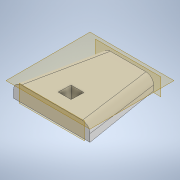
# Autodesk Inventor part: Botten
Saved by Autodesk Inventor 2021 (Build 250183000, 183)
## iProperties
Created: 2021-02-09
Part Number: Botten
Material: Generic
Document SubType Name: Modeling
Designer: marcu
Density: 1 g/cm^3
Appearance: Default
Author: marcu
## iProperties of the stored document _3DPrint.ipt
Created: 2021-02-16
Part Number: _3DPrint
Material: Generic
Document SubType Name: Modeling
Designer: marcu
Density: 1 g/cm^3
Appearance: Default
Author: marcu
Autodesk Inventor part; units mm, degrees
ref_plane "YZ Plane" through (0, 0, 0) normal (1, 0, 0) x (0, 1, 0)
ref_plane "XZ Plane" through (0, 0, 0) normal (0, 1, 0) x (-1, 0, 0)
ref_plane "XY Plane" through (0, 0, 0) normal (0, 0, 1) x (1, 0, 0)
sketch "Sketch6" plane through (0, 0, 0) normal (0, 0, 1) x (1, 0, 0)
  line L0 (0, 0) -> (100, 0)
  line L1 (100, 0) -> (100, 10)
  line L2 (85, 25) -> (15, 25)
  line L3 (0, 10) -> (0, 0)
  arc A0 (15, 25) -> (0, 10) centre (15, 10) ccw
  arc A1 (100, 10) -> (85, 25) centre (85, 10) ccw
  point P0 (100, 25)
  point P1 (0, 25)
  dimension "d18" = 100
  dimension "d19" = 25
  dimension "d20" = 15
  dimension "d21" = 15
  constraints: 8 end point, 4 point on circle, 4 point on line, 4 tangent, 2 centre point, 2 parallel, 1 horizontal, 1 perpendicular
  measures "d18" distance of point (100, 25) point (0, 25)
  measures "d19" distance of L0.end point (100, 25)
  measures "d20" radius of A0
  measures "d21" radius of A1
ref_plane "Work Plane1" through (85, 25, 0) normal (0, 0, 1) x (-1, 0, 0)
ref_plane "Work Plane2" through (85, 25, 150) normal (0, 0, 1) x (-1, 0, 0)
sketch "Sketch7" plane through (85, 25, 150) normal (0, 0, 1) x (-1, 0, 0)
  line L0 (110, 25) -> (-40, 25)
  line L1 (-40, 25) -> (-40, 10)
  line L2 (-25, -5) -> (95, -5)
  line L3 (110, 10) -> (110, 25)
  arc A0 (95, -5) -> (110, 10) centre (95, 10) ccw
  arc A1 (-40, 10) -> (-25, -5) centre (-25, 10) ccw
  point P0 (85, 25)
  point P1 (-40, -5)
  point P2 (110, -5)
  dimension "d23" = 30
  dimension "d24" = 150
  dimension "d25" = 25
  dimension "d26" = 15
  dimension "d27" = 15
  dimension "d42" = 0
  constraints: 8 end point, 4 point on circle, 4 point on line, 4 tangent, 2 centre point, 2 parallel, 1 horizontal, 1 perpendicular
  measures "d23" distance of L0.end point (-40, -5)
  measures "d24" distance of point (-40, -5) point (110, -5)
  measures "d25" distance from line of L3 point (85, 25)
  measures "d26" radius of A0
  measures "d27" radius of A1
  measures "d42" distance from line of point (85, 25) L0
loft "Loft1" add profiles "Sketch6", "Sketch7"
ref_plane "Work Plane3" through (110, 30, 150) normal (0, 1, 0) x (-1, 0, 0)
sketch "Sketch9" plane through (110, 30, 150) normal (0, 1, 0) x (-1, 0, 0)
  line L0 (72.75, -25) -> (47.25, -25)
  line L1 (47.25, -25) -> (47.25, -50.5)
  line L2 (47.25, -50.5) -> (72.75, -50.5)
  line L3 (72.75, -50.5) -> (72.75, -25)
  line L4 (0, 0) -> (120, 0) projected
  point P0 (110, -150)
  dimension "d45" = 25.5
  dimension "d46" = 25.5
  dimension "d47" = 25
  dimension "d48" = 47.25
  dimension "d49" = 47.25
  constraints: 8 end point, 2 parallel, 1 horizontal, 1 perpendicular
  measures "d45" distance of L1.end L2.end
  measures "d46" distance of L0.end L1.end
  measures "d47" distance between parallel lines of L4 L0
  measures "d48" distance from line of L4.end L3
  measures "d49" distance from line of L4.start L1
extrude "Extrusion2" cut sketch "Sketch9" against normal blind 25
body "Solid2"
